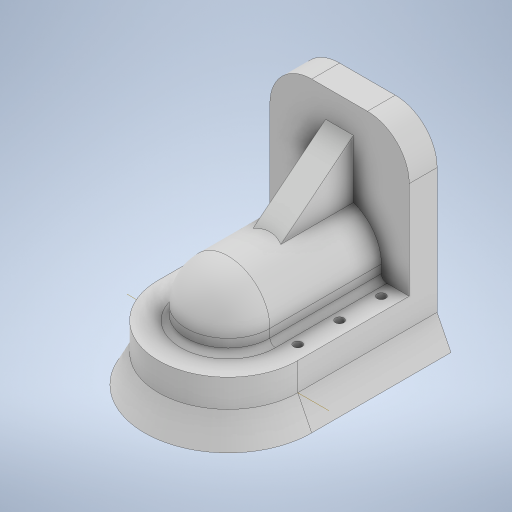
# Autodesk Inventor part: khurramf_Graphics4
Saved by Autodesk Inventor 2024 (Build 280153000, 153)
## iProperties
Created: 2023-10-27
Part Number: khurramf_Graphics4
Material: Generic
Document SubType Name: Modeling
Designer: furqa
Density: 1 g/cm^3
Appearance: Default
Author: furqa
Autodesk Inventor part; units mm, degrees
ref_plane "YZ Plane" through (0, 0, 0) normal (1, 0, 0) x (0, 1, 0)
ref_plane "XY Plane" through (0, 0, 0) normal (0, 0, 1) x (1, 0, 0)
sketch "Sketch1" plane through (0, 0, 0) normal (0, 1, 0) x (-1, 0, 0)
  line L0 (30, 0) -> (-30, 0)
  line L1 (-30, 0) -> (-30, 50)
  line L2 (30, 50) -> (30, 0)
  arc A0 (30, 50) -> (-30, 50) centre (0, 50) ccw
  point P0 (0, 0)
  point P1 (0, 0)
  constraints: 6 end point, 2 point on circle, 1 centre point, 1 horizontal, 1 midpoint, 1 parallel, 1 perpendicular, 1 tangent
ref_plane "Work Plane1" through (0, 10, 0) normal (0, 1, 0) x (-1, 0, 0)
sketch "Sketch5" plane through (0, 10, 0) normal (0, 1, 0) x (-1, 0, 0)
  line L0 (25, 0) -> (-25, 0)
  line L1 (-25, 0) -> (-25, 50)
  line L2 (-25, 50) -> (25, 50)
  line L3 (25, 50) -> (25, 0)
  arc A0 (25, 50) -> (-25, 50) centre (0, 50) ccw
  point P0 (0, 0)
  dimension "d11" = 50
  dimension "d12" = 50
  constraints: 8 end point, 2 parallel, 2 point on circle, 1 centre point, 1 horizontal, 1 perpendicular, 1 tangent
  measures "d11" distance of L1.end L2.end
  measures "d12" distance of L0.end L1.end
extrude "Extrusion1" add sketch "Sketch5" along normal blind 10
loft "Loft2" add profiles "Sketch1" section 2 edges at (25, 10, 25) (0, 10, 75) (-25, 10, 25) (0, 10, 0)
sketch "Sketch6" plane through (0, 0, 0) normal (1, 0, 0) x (0, 1, 0)
  line L0 (20, 0) -> (70, 0)
  line L1 (70, 0) -> (70, 10)
  line L2 (70, 10) -> (20, 10)
  line L3 (20, 10) -> (20, 0)
  point P0 (0, 0)
  dimension "d19" = 50
  dimension "d20" = 10
  constraints: 8 end point, 2 parallel, 1 horizontal, 1 perpendicular
  measures "d19" distance of L2.end L1.end
  measures "d20" distance of L1.end L0.end
extrude "Extrusion2" add sketch "Sketch6" along normal mid plane 50
fillet "Fillet1" radius 15 2 edges at (25, 70, 5) (-25, 70, 5)
sketch "Sketch7" plane through (0, 20, 0) normal (0, 1, 0) x (1, 0, 0)
  line L0 (25, -10) -> (-25, -10) projected
  line L1 (-15, -10) -> (15, -10)
  line L2 (15, -10) -> (15, -50)
  line L3 (15, -50) -> (-15, -50)
  line L4 (-15, -50) -> (-15, -10)
  circle A0 centre (-20, -15) radius 1.5
  circle A1 centre (-20, -30) radius 1.5
  circle A2 centre (-20, -45) radius 1.5
  line L5 (-10, -10) -> (-25, -10) projected
  line L6 (-25, -10) -> (-25, -50) projected
  line L7 (25, -50) -> (25, -10) projected
  point P0 (0, 0)
  point P1 (15, -10)
  point P2 (-17.5, -10)
  point P3 (-25, -30)
  dimension "d24" = 30
  dimension "d25" = 40
  dimension "d42" = 3
  dimension "d43" = 3
  dimension "d44" = 3
  dimension "d45" = 5
  dimension "d46" = 15
  dimension "d47" = 15
  dimension "d48" = 5
  dimension "d49" = 5
  dimension "d50" = 5
  dimension "d72" = 10
  dimension "d73" = 10
  constraints: 8 end point, 3 centre point, 2 midpoint, 2 parallel, 1 horizontal, 1 perpendicular, 1 point on line
  measures "d24" distance of L2.end L3.end
  measures "d25" distance of L1.end L2.end
  measures "d42" diameter of A0
  measures "d43" diameter of A1
  measures "d44" diameter of A2
  measures "d45" vertical distance of A0.centre point (-17.5, -10)
  measures "d46" distance of A0.centre A1.centre
  measures "d47" distance of A1.centre A2.centre
  measures "d48" distance of A1.centre point (-25, -30)
  measures "d49" distance from line of L6 A0.centre
  measures "d50" distance from line of L6 A2.centre
  measures "d72" distance between parallel lines of L4 L6
  measures "d73" distance between parallel lines of L7 L2
extrude "Extrusion3" add sketch "Sketch7" along normal blind 20 contours L2 L3 L4 L0
sketch "Sketch8" plane through (0, 20, 0) normal (0, 1, 0) x (1, 0, 0)
  line L0 (-15, -50) -> (15, -50) projected
  circle A0 centre (0, -50) radius 15
  point P0 (0, 0)
  constraints: 1 midpoint, 3 other
extrude "Extrusion4" add sketch "Sketch8" along normal blind 20 contours L0 A0 picked at (0.6027, -54.9635)
fillet "Fillet2" radius 15 3 edges at (0, 40, 65) (15, 40, 30) (-15, 40, 30)
fillet "Fillet3" radius 2 3 edges at (-15, 20, 30) (15, 20, 30) (0, 20, 65)
sketch "Sketch12" plane through (0, 0, 0) normal (1, 0, 0) x (0, 1, 0)
  line L0 (40, 10) -> (40, 50) projected
  line L1 (55, 10) -> (70, 10) projected
  line L2 (40, 35) -> (60, 10)
  point P0 (0, 0)
  constraints: 2 end point
extrude "Rib1" add sketch "Sketch12" along normal mid plane 10 rib yes fills toward (49.961, 22.4688) open curves L2
sketch "Sketch14" plane through (0, 20, 0) normal (0, 1, 0) x (1, 0, 0)
  circle A0 centre (-20, -15) radius 1.5
  circle A1 centre (-20, -30) radius 1.5
  circle A2 centre (-20, -44.9706) radius 1.5
  line L0 (-10, -10) -> (-25, -10) projected
  line L1 (-17, -10) -> (-17, -50) projected
  line L2 (-25, -10) -> (-25, -50) projected
  line L3 (-15, -10) -> (-15, -50) projected
  line L4 (-15, -50) -> (-15, -10) projected
  point P0 (0, 0)
  dimension "d51" = 3
  dimension "d52" = 3
  dimension "d53" = 3
  dimension "d74" = 5
  dimension "d75" = 5
  dimension "d76" = 5
  constraints: 3 centre point
  measures "d51" diameter of A0
  measures "d52" diameter of A1
  measures "d53" diameter of A2
  measures "d74" distance from line of L3 A2.centre
  measures "d75" distance from line of L4 A1.centre
  measures "d76" distance from line of L3 A0.centre
extrude "Extrusion5" cut sketch "Sketch14" against normal blind 20
sketch "Sketch15" plane through (0, 20, 0) normal (0, 1, 0) x (1, 0, 0)
  circle A0 centre (20, -15) radius 1.5
  circle A1 centre (20, -30) radius 1.5
  circle A2 centre (20, -45) radius 1.5
  line L0 (25, -10) -> (10, -10) projected
  line L1 (17, -50) -> (17, -10) projected
  line L2 (15, -10) -> (15, -50) projected
  point P0 (0, 0)
  point P1 (17, -30)
  point P2 (15, -30)
  dimension "d62" = 3
  dimension "d63" = 3
  dimension "d64" = 3
  dimension "d65" = 15
  dimension "d66" = 5
  dimension "d67" = 15
  dimension "d77" = 5
  dimension "d78" = 5
  dimension "d79" = 5
  constraints: 3 centre point, 2 midpoint
  measures "d62" diameter of A0
  measures "d63" diameter of A1
  measures "d64" diameter of A2
  measures "d65" distance of A1.centre A2.centre
  measures "d66" distance from line of A0.centre L0
  measures "d67" distance of A1.centre A0.centre
  measures "d77" distance from line of L2 A2.centre
  measures "d78" distance of point (15, -30) A1.centre
  measures "d79" distance from line of L2 A0.centre
extrude "Extrusion6" cut sketch "Sketch15" against normal blind 20
sketch "Sketch18" plane through (30, 0, 0) normal (0, 0, -1) x (-1, 0, 0)
  line L0 (60, 0) -> (0, 0) projected
  line L1 (15, 0) -> (45, 0)
  line L2 (45, 0) -> (45, 10)
  line L3 (15, 10) -> (15, 0)
  arc A0 (45, 10) -> (15, 10) centre (30, 10) ccw
  point P0 (30, 0)
  point P1 (30, 0)
  point P2 (30, 0)
  constraints: 6 end point, 2 midpoint, 2 point on circle, 1 centre point, 1 horizontal, 1 parallel, 1 perpendicular, 1 point on line, 1 tangent
extrude "Extrusion7" cut sketch "Sketch18" against normal blind 50
sketch "Sketch24" plane through (30, 0, 50) normal (0, 0, -1) x (-1, 0, 0)
  line L0 (15, 0) -> (15, 10) projected
  line L1 (45, 10) -> (45, 0) projected
  point P0 (30, 0)
sketch "Sketch25" plane through (30, 0, 50) normal (0, 0, -1) x (-1, 0, 0)
  line L0 (55, 10) -> (5, 10) projected
  arc A0 (45, 10) -> (15, 10) centre (30, 10) ccw
  line L1 (45, 25) -> (15, 25) projected
  point P0 (30, 0)
  constraints: 2 point on circle, 2 point on line, 1 centre point, 1 midpoint, 1 tangent
sketch "Sketch26" plane through (0, 0, 50) normal (0, -1, 0) x (1, 0, 0)
  line L0 (15, 0) -> (-15, 0) projected
  arc A0 (15, 0) -> (-15, 0) centre (0, 0) ccw
  point P0 (0, -50)
  constraints: 2 end point, 2 point on circle, 1 centre point, 1 midpoint
extrude "Extrusion8" cut sketch "Sketch26" against normal blind 10
revolve "Revolution1" cut sketch "Sketch25" angle 360 about axis through (-25, 10, 50) along (1, 0, 0)
body "Solid2"
